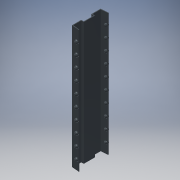
# Autodesk Inventor part: slider_SSRN3618
Saved by Autodesk Inventor 2016 (Build 200138000, 138)
## iProperties
Category: PARTsolutions
Company: MISUMI
Created: 2016-11-23
Part Number: slider_SSRN3618
Catalog Web Link: www.cadenas.de
Description: slider_ssrn36-Slide Rails - Stainles Steel - Two - Step Slide Rails
Vendor: MISUMI
Document SubType Name: Modeling
Designer: psAdmin
Manufacturer: MISUMI
Mass: 33.7161 g
Surface Area: 129.132 cm^2
Volume: 4.71554 cm^3
Density: 7.15 g/cm^3
Material: 鉄 灰色
Appearance: 鉄 灰色
PSOL_IDENT_0: {$CADENAS_DATA\23d-libs\misumi\metric\07_slide_rails\ssrn36_series\ssrn36_slider.prj},172 {VTYP=3D},
PSOL_IDENT_1: {NB=slider_SSRN3618},{LINA=slider_SSRN3618},{NN=slider_ssrn36},{DATE=17.06.2016 05:46:12},{GEOMDATE=
PSOL_IDENT_2: 16.03.2005},{VERSION=},{LINEID=10},{LINESUBID=-1},{WBVAR=NO}  {NB=slider_SSRN3618},{LINA=slider_SSRN
PSOL_IDENT_3: 3618},{KT=DUMMY},{PN=SSRN3618},{TYPE=SSRN3618},{MATR=Rail 304 Stainless Steel},{MATB=Ball 440C Stain
PSOL_IDENT_4: less Steel},{NO=18},{RL=457.2},{TD=330.2},{A=203.2},{B=304.8},{C=406.4},{D=212.7},{E=301.6},{F=412.7
PSOL_IDENT_5: },{G=425.4},{RLD=402},{NOB=10}
NN: slider_ssrn36
NT: Slide Rails - Stainles Steel - Two - Step Slide Rails
NB: slider_SSRN3618
NBSYN: slider_$PN.
LINA: slider_SSRN3618
MATR: Rail 304 Stainless Steel
MATB: Ball 440C Stainless Steel
NO: 18
SUPPLIER: MISUMI
ARTICLENO: slider_SSRN3618
BOMINFO: slider_SSRN3618
CREATOR: CADENAS GmbH
Title: slider_SSRN3618
Author: Cadenas PARTsolutions
Comments: Slide Rails - Stainles Steel - Two - Step Slide Rails
Autodesk Inventor part; units mm, degrees
sketch "Sketch_1" plane through (0, 0, 0) normal (0, 0, 1) x (1, 0, 0)
  line L0 (1, 2.8443) -> (8.8, 2.1619)
  line L1 (8.8, 2.1619) -> (8.8, 2.8646)
  line L2 (8.8, 2.8646) -> (1.7, 3.4857)
  line L3 (1.7, 3.4857) -> (1.7, 11.7169)
  line L4 (1.7, 11.7169) -> (4.3, 11.9444)
  line L5 (4.3, 11.9444) -> (4.3, 23.3556)
  line L6 (4.3, 23.3556) -> (1.7, 23.5831)
  line L7 (1.7, 23.5831) -> (1.7, 31.8143)
  line L8 (1.7, 31.8143) -> (8.8, 32.4354)
  line L9 (8.8, 32.4354) -> (8.8, 33.1381)
  line L10 (8.8, 33.1381) -> (1, 32.4557)
  line L11 (1, 32.4557) -> (1, 22.9444)
  line L12 (1, 22.9444) -> (3.6, 22.7169)
  line L13 (3.6, 22.7169) -> (3.6, 12.5831)
  line L14 (3.6, 12.5831) -> (1, 12.3556)
  line L15 (1, 12.3556) -> (1, 2.8443)
  constraints: 32 end point
extrude "Extrusion1" add sketch "Sketch_1" along normal blind 127
sketch "Sketch_2" plane through (0, 2.35, 0) normal (0, 1, 0) x (1, 0, 0)
  line L0 (6.65, -11.85) -> (6.65, -8.15)
  arc A0 (6.65, -11.85) -> (6.65, -8.15) centre (6.65, -10) ccw
  line L1 (6.65, -11.85) -> (6.65, -8.15)
  constraints: 4 end point, 2 point on circle, 1 centre point
revolve "Revolution1" add sketch "Sketch_2" angle 360 about axis through (6.65, 2.35, 11.85) along (0, 0, 1)
pattern_linear "Rectangular Pattern1" count 10 spacing 11.7 along (0, 0, 1) of "Revolution1"
sketch "Sketch_4" plane through (0, 32.95, 0) normal (0, 1, 0) x (1, 0, 0)
  line L0 (6.65, -11.85) -> (6.65, -8.15)
  arc A0 (6.65, -11.85) -> (6.65, -8.15) centre (6.65, -10) ccw
  line L1 (6.65, -11.85) -> (6.65, -8.15)
  constraints: 4 end point, 2 point on circle, 1 centre point
revolve "Revolution2" add sketch "Sketch_4" angle 360 about axis through (6.65, 32.95, 11.85) along (0, 0, 1)
pattern_linear "Rectangular Pattern2" count 10 spacing 11.7 along (0, 0, 1) of "Revolution2"
ref_plane "to_rail_XY" through (9.5, 17.65, 63.5) normal (0, 0, 1) x (1, 0, 0)
ref_plane "to_rail_YZ" through (9.5, 17.65, 63.5) normal (1, 0, 0) x (0, 1, 0)
ref_plane "to_rail_ZX" through (9.5, 17.65, 63.5) normal (0, 1, 0) x (0, 0, 1)
body "Solid1"
